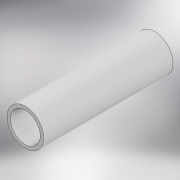
# Autodesk Inventor part: Tubo4
Saved by Autodesk Inventor 2021 (Build 250183000, 183)
## iProperties
Created: 2024-02-21
Part Number: Tubo4
Material: Generic
Document SubType Name: Modeling
Designer: Martin
Density: 1 g/cm^3
Appearance: Default
Author: Martin
Autodesk Inventor part; units mm, degrees
ref_plane "YZ Plane" through (0, 0, 0) normal (1, 0, 0) x (0, 1, 0)
ref_plane "XZ Plane" through (0, 0, 0) normal (0, 1, 0) x (-1, 0, 0)
ref_plane "XY Plane" through (0, 0, 0) normal (0, 0, 1) x (1, 0, 0)
sketch "Sketch1" plane through (0, 0, 0) normal (0, 0, 1) x (1, 0, 0)
  circle A0 centre (0, 0) radius 7.8
  circle A1 centre (0, 0) radius 6.35
  dimension "d0" = 15.6
  dimension "d1" = 12.7
  constraints: 2 centre point, 2 coincident
  measures "d0" diameter of A0
  measures "d1" diameter of A1
extrude "Extrusion1" add sketch "Sketch1" along normal blind 55
body "Solid1"
